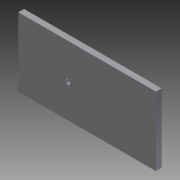
# Autodesk Inventor part: tiltBoxRightSide
Saved by Autodesk Inventor 2012 (Build 160160000, 160)
## iProperties
Created: 2014-06-13
Part Number: tiltBoxRightSide
Material: Default
Document SubType Name: Modeling
Designer: Byron
Density: 1 g/cm^3
Author: Byron
Autodesk Inventor part; units mm, degrees
ref_plane "YZ Plane" through (0, 0, 0) normal (1, 0, 0) x (0, 1, 0)
ref_plane "XZ Plane" through (0, 0, 0) normal (0, 1, 0) x (-1, 0, 0)
ref_plane "XY Plane" through (0, 0, 0) normal (0, 0, 1) x (1, 0, 0)
sketch "Sketch1" plane through (0, 0, 0) normal (0, 0, 1) x (1, 0, 0)
  line L0 (-106.0077, -14.9233) -> (-106.0077, -35.8767) projected
  line L1 (-106.0077, -25.4) -> (-42.6709, -25.4) construction
  line L2 (-84.8276, 0) -> (-110.2276, 0) construction
  line L3 (-97.5276, 0) -> (-97.5276, -25.4) construction
  line L4 (0, 6.35) -> (-152.4, 6.35) projected
  line L5 (-152.4, 0) -> (-152.4, 6.35) projected
  line L6 (0, 0) -> (-152.4, 0) projected
  line L7 (0, 0) -> (0, 6.35) projected
  line L8 (0, 6.35) -> (0, -101.238) construction
  line L9 (-152.4, 6.35) -> (-152.4, -106.3587) construction
  line L10 (0, -61.9376) -> (-152.4, -61.9376)
  line L11 (-152.4, -61.9376) -> (-152.4, 14.2624)
  line L12 (-152.4, 14.2624) -> (0, 14.2624)
  line L13 (0, 14.2624) -> (0, -61.9376)
  circle A0 centre (-97.5276, -25.4) radius 2.5
  dimension "d2" = 5
  dimension "d5" = 76.2
  constraints: 16 end point, 3 coincident, 3 parallel, 3 perpendicular, 2 horizontal, 2 midpoint, 2 point on line, 1 centre point, 1 collinear, 2 other
  measures "d2" diameter of A0
  measures "d5" distance of L10.end L11.end
extrude "Extrusion2" add sketch "Sketch1" along normal blind 6.35
body "Solid2"
